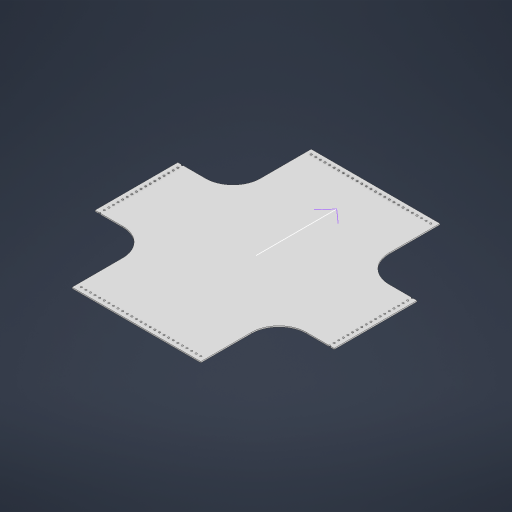
# Autodesk Inventor part: Belly_Pan
Saved by Autodesk Inventor 2024.2 (Build 282272000, 272)
## iProperties
Created: 2024-07-20
Part Number: Belly_Pan
Material: Generic
Document SubType Name: Modeling
Designer: Rocky
Density: 1 g/cm^3
Appearance: Default
Author: Rocky
Autodesk Inventor part; units mm, degrees
ref_plane "YZ Plane" through (0, 0, 0) normal (1, 0, 0) x (0, 1, 0)
ref_plane "XZ Plane" through (0, 0, 0) normal (0, 1, 0) x (-1, 0, 0)
ref_plane "XY Plane" through (0, 0, 0) normal (0, 0, 1) x (1, 0, 0)
sketch "Base" plane through (0, 0, 0) normal (0, 1, 0) x (-1, 0, 0)
  line L0 (330.2, 330.2) -> (-330.2, 330.2)
  line L1 (-330.2, 330.2) -> (-330.2, -330.2)
  line L2 (-330.2, -330.2) -> (330.2, -330.2)
  line L3 (330.2, -330.2) -> (330.2, 330.2)
  line L4 (330.2, 330.2) -> (-330.2, -330.2) construction
  line L5 (-330.2, 330.2) -> (330.2, -330.2) construction
  circle A0 centre (317.5, 165.1) radius 2.4892
  circle A1 centre (317.5, 152.4) radius 2.4892
  circle A2 centre (317.5, 139.7) radius 2.4892
  circle A3 centre (317.5, 127) radius 2.4892
  circle A4 centre (317.5, 114.3) radius 2.4892
  circle A5 centre (317.5, 101.6) radius 2.4892
  circle A6 centre (317.5, 88.9) radius 2.4892
  circle A7 centre (317.5, 76.2) radius 2.4892
  circle A8 centre (317.5, 63.5) radius 2.4892
  circle A9 centre (317.5, 50.8) radius 2.4892
  circle A10 centre (317.5, 38.1) radius 2.4892
  circle A11 centre (317.5, 25.4) radius 2.4892
  circle A12 centre (317.5, 12.7) radius 2.4892
  circle A13 centre (317.5, 0) radius 2.4892
  circle A14 centre (317.5, -12.7) radius 2.4892
  circle A15 centre (317.5, -25.4) radius 2.4892
  circle A16 centre (317.5, -38.1) radius 2.4892
  circle A17 centre (317.5, -50.8) radius 2.4892
  circle A18 centre (317.5, -63.5) radius 2.4892
  circle A19 centre (317.5, -76.2) radius 2.4892
  circle A20 centre (317.5, -88.9) radius 2.4892
  circle A21 centre (317.5, -101.6) radius 2.4892
  circle A22 centre (317.5, -114.3) radius 2.4892
  circle A23 centre (317.5, -127) radius 2.4892
  circle A24 centre (317.5, -139.7) radius 2.4892
  circle A25 centre (317.5, -152.4) radius 2.4892
  circle A26 centre (317.5, -165.1) radius 2.4892
  line L6 (330.2, 177.8) -> (304.8, 177.8)
  line L7 (177.8, 330.2) -> (177.8, 304.8)
  circle A27 centre (304.8, 304.8) radius 127 construction
  line L8 (304.8, 304.8) -> (177.8, 304.8) construction
  line L9 (304.8, 177.8) -> (304.8, 304.8) construction
  arc A28 (177.8, 304.8) -> (304.8, 177.8) centre (304.8, 304.8) ccw
  arc A29 (-304.8, 177.8) -> (-177.8, 304.8) centre (-304.8, 304.8) ccw
  line L10 (-177.8, 330.2) -> (-177.8, 304.8)
  line L11 (-330.2, 177.8) -> (-304.8, 177.8)
  arc A30 (-177.8, -304.8) -> (-304.8, -177.8) centre (-304.8, -304.8) ccw
  line L12 (-330.2, -177.8) -> (-304.8, -177.8)
  line L13 (-177.8, -330.2) -> (-177.8, -304.8)
  arc A31 (304.8, -177.8) -> (177.8, -304.8) centre (304.8, -304.8) ccw
  line L14 (177.8, -330.2) -> (177.8, -304.8)
  line L15 (330.2, -177.8) -> (304.8, -177.8)
  circle A32 centre (0, 317.5) radius 2.4892
  circle A33 centre (12.7, 317.5) radius 2.4892
  circle A34 centre (25.4, 317.5) radius 2.4892
  circle A35 centre (38.1, 317.5) radius 2.4892
  circle A36 centre (50.8, 317.5) radius 2.4892
  circle A37 centre (63.5, 317.5) radius 2.4892
  circle A38 centre (88.9, 317.5) radius 2.4892
  circle A39 centre (76.2, 317.5) radius 2.4892
  circle A40 centre (101.6, 317.5) radius 2.4892
  circle A41 centre (114.3, 317.5) radius 2.4892
  circle A42 centre (127, 317.5) radius 2.4892
  circle A43 centre (139.7, 317.5) radius 2.4892
  circle A44 centre (152.4, 317.5) radius 2.4892
  circle A45 centre (165.1, 317.5) radius 2.4892
  circle A46 centre (-165.1, 317.5) radius 2.4892
  circle A47 centre (-152.4, 317.5) radius 2.4892
  circle A48 centre (-139.7, 317.5) radius 2.4892
  circle A49 centre (-127, 317.5) radius 2.4892
  circle A50 centre (-114.3, 317.5) radius 2.4892
  circle A51 centre (-12.7, 317.5) radius 2.4892
  circle A52 centre (-25.4, 317.5) radius 2.4892
  circle A53 centre (-38.1, 317.5) radius 2.4892
  circle A54 centre (-50.8, 317.5) radius 2.4892
  circle A55 centre (-63.5, 317.5) radius 2.4892
  circle A56 centre (-88.9, 317.5) radius 2.4892
  circle A57 centre (-101.6, 317.5) radius 2.4892
  circle A58 centre (-76.2, 317.5) radius 2.4892
  circle A59 centre (-317.5, 0) radius 2.4892
  circle A60 centre (-317.5, 12.7) radius 2.4892
  circle A61 centre (-317.5, 25.4) radius 2.4892
  circle A62 centre (-317.5, 38.1) radius 2.4892
  circle A63 centre (-317.5, 50.8) radius 2.4892
  circle A64 centre (-317.5, 63.5) radius 2.4892
  circle A65 centre (-317.5, 88.9) radius 2.4892
  circle A66 centre (-317.5, 76.2) radius 2.4892
  circle A67 centre (-317.5, 101.6) radius 2.4892
  circle A68 centre (-317.5, 114.3) radius 2.4892
  circle A69 centre (-317.5, 127) radius 2.4892
  circle A70 centre (-317.5, 139.7) radius 2.4892
  circle A71 centre (-317.5, 152.4) radius 2.4892
  circle A72 centre (-317.5, 165.1) radius 2.4892
  circle A73 centre (-317.5, -165.1) radius 2.4892
  circle A74 centre (-317.5, -152.4) radius 2.4892
  circle A75 centre (-317.5, -139.7) radius 2.4892
  circle A76 centre (-317.5, -127) radius 2.4892
  circle A77 centre (-317.5, -114.3) radius 2.4892
  circle A78 centre (-317.5, -12.7) radius 2.4892
  circle A79 centre (-317.5, -25.4) radius 2.4892
  circle A80 centre (-317.5, -38.1) radius 2.4892
  circle A81 centre (-317.5, -50.8) radius 2.4892
  circle A82 centre (-317.5, -63.5) radius 2.4892
  circle A83 centre (-317.5, -88.9) radius 2.4892
  circle A84 centre (-317.5, -101.6) radius 2.4892
  circle A85 centre (-317.5, -76.2) radius 2.4892
  circle A86 centre (0, -317.5) radius 2.4892
  circle A87 centre (-12.7, -317.5) radius 2.4892
  circle A88 centre (-25.4, -317.5) radius 2.4892
  circle A89 centre (-38.1, -317.5) radius 2.4892
  circle A90 centre (-50.8, -317.5) radius 2.4892
  circle A91 centre (-63.5, -317.5) radius 2.4892
  circle A92 centre (-88.9, -317.5) radius 2.4892
  circle A93 centre (-76.2, -317.5) radius 2.4892
  circle A94 centre (-101.6, -317.5) radius 2.4892
  circle A95 centre (-114.3, -317.5) radius 2.4892
  circle A96 centre (-127, -317.5) radius 2.4892
  circle A97 centre (-139.7, -317.5) radius 2.4892
  circle A98 centre (-152.4, -317.5) radius 2.4892
  circle A99 centre (-165.1, -317.5) radius 2.4892
  circle A100 centre (165.1, -317.5) radius 2.4892
  circle A101 centre (152.4, -317.5) radius 2.4892
  circle A102 centre (139.7, -317.5) radius 2.4892
  circle A103 centre (127, -317.5) radius 2.4892
  circle A104 centre (114.3, -317.5) radius 2.4892
  circle A105 centre (12.7, -317.5) radius 2.4892
  circle A106 centre (25.4, -317.5) radius 2.4892
  circle A107 centre (38.1, -317.5) radius 2.4892
  circle A108 centre (50.8, -317.5) radius 2.4892
  circle A109 centre (63.5, -317.5) radius 2.4892
  circle A110 centre (88.9, -317.5) radius 2.4892
  circle A111 centre (101.6, -317.5) radius 2.4892
  circle A112 centre (76.2, -317.5) radius 2.4892
  point P0 (0, 0)
  point P1 (304.8, 177.8)
  point P2 (-177.8, 330.2)
  point P3 (-177.8, 304.8)
  point P4 (-304.8, 177.8)
  point P5 (-330.2, -177.8)
  point P6 (-304.8, -177.8)
  point P7 (-177.8, -304.8)
  point P8 (177.8, -330.2)
  point P9 (177.8, -304.8)
  point P10 (304.8, -177.8)
  point P11 (177.8, 330.2)
  point P12 (-330.2, 177.8)
  point P13 (-177.8, -330.2)
  dimension "d0" = 660.4
  dimension "d1" = 660.4
  dimension "d2" = 165.1
  dimension "d3" = 12.7
  dimension "d4" = 4.9784
  dimension "d7" = 12.7
  dimension "d16" = 152.4
  dimension "d17" = 152.4
  dimension "d18" = 25.4
  dimension "d19" = 25.4
  dimension "d20" = 90
  dimension "d21" = 90
  dimension "d22" = 90
  dimension "d25" = 360
  dimension "d31" = 360
  constraints: 113 centre point, 32 end point, 10 point on circle, 8 coincident, 4 point on line, 2 horizontal, 2 midpoint, 2 parallel, 2 vertical, 1 perpendicular, 314 other
  measures "d0" distance of L2.end L1.end
  measures "d1" distance of L1.end L0.end
  measures "d2" distance from line of L0 point (317.5, 165.1)
  measures "d3" distance from line of L3 point (317.5, 165.1)
  measures "d4" diameter of A0
  measures "d7" distance of A0.centre A1.centre
  measures "d16" distance of L0.start L6.start
  measures "d17" distance of L7.start L0.start
  measures "d18" distance of L6.start L6.end
  measures "d19" distance of L7.start L7.end
  measures "d20" angle of L0 L7
  measures "d21" angle of L3 L6
  measures "d22" angle of L8 L9
extrude "Extrusion1" add sketch "Base" along normal blind 3.175 contours L7 A28 L6 L3 L15 A31 L14 L2 L13 A30 L12 L1 L11 A29 L10 L0
sketch "Sketch2" plane through (0, 3.175, 0) normal (0, 1, 0) x (1, 0, 0)
  line L0 (0, 0) -> (0, 222.393)
  line L1 (0, 222.393) -> (36.8995, 189.6171)
  line L2 (0, 222.393) -> (-29.1132, 189.6171)
  constraints: 6 end point, 1 vertical
sketch "Sketch5" plane through (0, 3.175, 0) normal (0, 1, 0) x (1, 0, 0)
  line L0 (-330.2, 177.8) -> (-330.2, -177.8) projected
  line L1 (177.8, 330.2) -> (-177.8, 330.2) projected
  line L2 (330.2, -177.8) -> (330.2, 177.8) projected
  line L3 (-177.8, -330.2) -> (177.8, -330.2) projected
  line L4 (-177.8, 330.2) -> (-330.2, 330.2)
  line L5 (-330.2, 330.2) -> (-330.2, 114.3)
  line L6 (-330.2, 114.3) -> (-254, 114.3)
  line L7 (-177.8, 190.5) -> (-177.8, 330.2)
  line L8 (177.8, 330.2) -> (330.2, 330.2)
  line L9 (330.2, 330.2) -> (330.2, 114.3)
  line L10 (330.2, 114.3) -> (254, 114.3)
  line L11 (177.8, 190.5) -> (177.8, 330.2)
  line L12 (-330.2, -114.3) -> (-254, -114.3)
  line L13 (-177.8, -190.5) -> (-177.8, -330.2)
  line L14 (-177.8, -330.2) -> (-330.2, -330.2)
  line L15 (-330.2, -330.2) -> (-330.2, -114.3)
  line L16 (177.8, -330.2) -> (177.8, -304.8) projected
  line L17 (177.8, -330.2) -> (330.2, -330.2)
  line L18 (330.2, -330.2) -> (330.2, -114.3)
  line L19 (330.2, -114.3) -> (254, -114.3)
  line L20 (177.8, -190.5) -> (177.8, -330.2)
  arc A0 (-254, 114.3) -> (-177.8, 190.5) centre (-254, 190.5) ccw
  arc A1 (177.8, 190.5) -> (254, 114.3) centre (254, 190.5) ccw
  arc A2 (254, -114.3) -> (177.8, -190.5) centre (254, -190.5) ccw
  arc A3 (-177.8, -190.5) -> (-254, -114.3) centre (-254, -190.5) ccw
  line L21 (-177.8, -304.8) -> (-177.8, -330.2) projected
  line L22 (-177.8, -330.2) -> (177.8, -330.2) projected
  line L23 (177.8, -330.2) -> (177.8, -304.8) projected
  arc A4 (304.8, -177.8) -> (177.8, -304.8) centre (304.8, -304.8) ccw projected
  line L24 (304.8, -177.8) -> (330.2, -177.8) projected
  line L25 (330.2, -177.8) -> (330.2, 177.8) projected
  line L26 (330.2, 177.8) -> (304.8, 177.8) projected
  arc A5 (177.8, 304.8) -> (304.8, 177.8) centre (304.8, 304.8) ccw projected
  line L27 (177.8, 304.8) -> (177.8, 330.2) projected
  line L28 (177.8, 330.2) -> (-177.8, 330.2) projected
  line L29 (-177.8, 330.2) -> (-177.8, 304.8) projected
  arc A6 (-304.8, 177.8) -> (-177.8, 304.8) centre (-304.8, 304.8) ccw projected
  line L30 (-304.8, 177.8) -> (-330.2, 177.8) projected
  line L31 (-330.2, 177.8) -> (-330.2, -177.8) projected
  line L32 (-330.2, -177.8) -> (-304.8, -177.8) projected
  arc A7 (-177.8, -304.8) -> (-304.8, -177.8) centre (-304.8, -304.8) ccw projected
  circle A8 centre (-76.2, 317.5) radius 2.4892 projected
  circle A9 centre (-88.9, 317.5) radius 2.4892 projected
  circle A10 centre (-50.8, 317.5) radius 2.4892 projected
  circle A11 centre (-25.4, 317.5) radius 2.4892 projected
  circle A12 centre (-114.3, 317.5) radius 2.4892 projected
  circle A13 centre (-139.7, 317.5) radius 2.4892 projected
  circle A14 centre (-165.1, 317.5) radius 2.4892 projected
  circle A15 centre (152.4, 317.5) radius 2.4892 projected
  circle A16 centre (127, 317.5) radius 2.4892 projected
  circle A17 centre (101.6, 317.5) radius 2.4892 projected
  circle A18 centre (88.9, 317.5) radius 2.4892 projected
  circle A19 centre (50.8, 317.5) radius 2.4892 projected
  circle A20 centre (25.4, 317.5) radius 2.4892 projected
  circle A21 centre (0, 317.5) radius 2.4892 projected
  circle A22 centre (317.5, 101.6) radius 2.4892 projected
  circle A23 centre (317.5, 63.5) radius 2.4892 projected
  circle A24 centre (317.5, 38.1) radius 2.4892 projected
  circle A25 centre (317.5, 12.7) radius 2.4892 projected
  circle A26 centre (317.5, 127) radius 2.4892 projected
  circle A27 centre (317.5, 152.4) radius 2.4892 projected
  circle A28 centre (317.5, -165.1) radius 2.4892 projected
  circle A29 centre (317.5, -139.7) radius 2.4892 projected
  circle A30 centre (317.5, -114.3) radius 2.4892 projected
  circle A31 centre (317.5, -76.2) radius 2.4892 projected
  circle A32 centre (317.5, -63.5) radius 2.4892 projected
  circle A33 centre (317.5, -38.1) radius 2.4892 projected
  circle A34 centre (317.5, -12.7) radius 2.4892 projected
  circle A35 centre (76.2, -317.5) radius 2.4892 projected
  circle A36 centre (88.9, -317.5) radius 2.4892 projected
  circle A37 centre (50.8, -317.5) radius 2.4892 projected
  circle A38 centre (25.4, -317.5) radius 2.4892 projected
  circle A39 centre (114.3, -317.5) radius 2.4892 projected
  circle A40 centre (139.7, -317.5) radius 2.4892 projected
  circle A41 centre (165.1, -317.5) radius 2.4892 projected
  circle A42 centre (-152.4, -317.5) radius 2.4892 projected
  circle A43 centre (-127, -317.5) radius 2.4892 projected
  circle A44 centre (-101.6, -317.5) radius 2.4892 projected
  circle A45 centre (-88.9, -317.5) radius 2.4892 projected
  circle A46 centre (-50.8, -317.5) radius 2.4892 projected
  circle A47 centre (-25.4, -317.5) radius 2.4892 projected
  circle A48 centre (0, -317.5) radius 2.4892 projected
  circle A49 centre (-317.5, 152.4) radius 2.4892 projected
  circle A50 centre (-317.5, 127) radius 2.4892 projected
  circle A51 centre (-317.5, 101.6) radius 2.4892 projected
  circle A52 centre (-317.5, 76.2) radius 2.4892 projected
  circle A53 centre (-317.5, 50.8) radius 2.4892 projected
  circle A54 centre (-317.5, 25.4) radius 2.4892 projected
  circle A55 centre (-317.5, 0) radius 2.4892 projected
  circle A56 centre (-317.5, -25.4) radius 2.4892 projected
  circle A57 centre (-317.5, -50.8) radius 2.4892 projected
  circle A58 centre (-317.5, -76.2) radius 2.4892 projected
  circle A59 centre (-317.5, -88.9) radius 2.4892 projected
  circle A60 centre (-317.5, -101.6) radius 2.4892 projected
  circle A61 centre (-317.5, -114.3) radius 2.4892 projected
  circle A62 centre (-317.5, -127) radius 2.4892 projected
  circle A63 centre (-317.5, -139.7) radius 2.4892 projected
  circle A64 centre (-317.5, -152.4) radius 2.4892 projected
  circle A65 centre (-317.5, -165.1) radius 2.4892 projected
  circle A66 centre (-317.5, -63.5) radius 2.4892 projected
  circle A67 centre (-317.5, -38.1) radius 2.4892 projected
  circle A68 centre (-317.5, -12.7) radius 2.4892 projected
  circle A69 centre (-317.5, 12.7) radius 2.4892 projected
  circle A70 centre (-317.5, 38.1) radius 2.4892 projected
  circle A71 centre (-317.5, 63.5) radius 2.4892 projected
  circle A72 centre (-317.5, 88.9) radius 2.4892 projected
  circle A73 centre (-317.5, 114.3) radius 2.4892 projected
  circle A74 centre (-317.5, 139.7) radius 2.4892 projected
  circle A75 centre (-317.5, 165.1) radius 2.4892 projected
  circle A76 centre (-12.7, -317.5) radius 2.4892 projected
  circle A77 centre (-38.1, -317.5) radius 2.4892 projected
  circle A78 centre (-63.5, -317.5) radius 2.4892 projected
  circle A79 centre (-76.2, -317.5) radius 2.4892 projected
  circle A80 centre (-114.3, -317.5) radius 2.4892 projected
  circle A81 centre (-139.7, -317.5) radius 2.4892 projected
  circle A82 centre (-165.1, -317.5) radius 2.4892 projected
  circle A83 centre (152.4, -317.5) radius 2.4892 projected
  circle A84 centre (127, -317.5) radius 2.4892 projected
  circle A85 centre (12.7, -317.5) radius 2.4892 projected
  circle A86 centre (38.1, -317.5) radius 2.4892 projected
  circle A87 centre (63.5, -317.5) radius 2.4892 projected
  circle A88 centre (101.6, -317.5) radius 2.4892 projected
  circle A89 centre (317.5, 0) radius 2.4892 projected
  circle A90 centre (317.5, -25.4) radius 2.4892 projected
  circle A91 centre (317.5, -50.8) radius 2.4892 projected
  circle A92 centre (317.5, -88.9) radius 2.4892 projected
  circle A93 centre (317.5, -101.6) radius 2.4892 projected
  circle A94 centre (317.5, -127) radius 2.4892 projected
  circle A95 centre (317.5, -152.4) radius 2.4892 projected
  circle A96 centre (317.5, 165.1) radius 2.4892 projected
  circle A97 centre (317.5, 139.7) radius 2.4892 projected
  circle A98 centre (317.5, 114.3) radius 2.4892 projected
  circle A99 centre (317.5, 25.4) radius 2.4892 projected
  circle A100 centre (317.5, 50.8) radius 2.4892 projected
  circle A101 centre (317.5, 88.9) radius 2.4892 projected
  circle A102 centre (317.5, 76.2) radius 2.4892 projected
  circle A103 centre (12.7, 317.5) radius 2.4892 projected
  circle A104 centre (38.1, 317.5) radius 2.4892 projected
  circle A105 centre (63.5, 317.5) radius 2.4892 projected
  circle A106 centre (76.2, 317.5) radius 2.4892 projected
  circle A107 centre (114.3, 317.5) radius 2.4892 projected
  circle A108 centre (139.7, 317.5) radius 2.4892 projected
  circle A109 centre (165.1, 317.5) radius 2.4892 projected
  circle A110 centre (-152.4, 317.5) radius 2.4892 projected
  circle A111 centre (-127, 317.5) radius 2.4892 projected
  circle A112 centre (-12.7, 317.5) radius 2.4892 projected
  circle A113 centre (-38.1, 317.5) radius 2.4892 projected
  circle A114 centre (-63.5, 317.5) radius 2.4892 projected
  circle A115 centre (-101.6, 317.5) radius 2.4892 projected
  point P0 (0, 0)
  point P1 (-315.0108, -114.3)
  point P2 (-319.9892, -114.3)
  point P3 (319.9892, -114.3)
  point P4 (315.0108, -114.3)
  point P5 (315.0108, 114.3)
  point P6 (319.9892, 114.3)
  point P7 (330.2, 177.8)
  point P8 (177.8, 304.8)
  point P9 (-319.9892, 114.3)
  point P10 (-315.0108, 114.3)
  dimension "d46" = 215.9
  dimension "d47" = 215.9
  dimension "d48" = 215.9
  dimension "d49" = 215.9
  dimension "d50" = 76.2
  dimension "d51" = 76.2
  constraints: 32 end point, 8 parallel, 8 point on circle, 8 tangent, 4 centre point, 4 horizontal, 4 perpendicular, 4 point on line, 2 equal radius
  measures "d46" distance from line of L5.end L1
  measures "d47" distance from line of L1 L9.end
  measures "d48" distance from line of L3 L12.start
  measures "d49" distance between parallel lines of L17 L19
  measures "d50" radius of A0
  measures "d51" radius of A1
extrude "Extrusion3" cut sketch "Sketch5" against normal blind 25.4 contours L30 A6 L7 A0 L6 A73 L0 | L12 A61 A3 L13 A7 L32 L0 | A5 L26 L2 L10 A98 A1 L11 | L20 A2 L19 A30 L2 L24 A4
body "Solid1"
